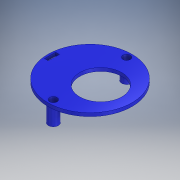
# Autodesk Inventor part: plate_r1
Saved by Autodesk Inventor 2018 (Build 220112000, 112)
## iProperties
Created: 2019-05-28
Part Number: plate_r1
Material: Generic
Document SubType Name: Modeling
Designer: Koki
Density: 1 g/cm^3
Appearance: Blue - Wall Paint - Glossy
Author: Koki
Autodesk Inventor part; units mm, degrees
ref_plane "YZ Plane" through (0, 0, 0) normal (1, 0, 0) x (0, 1, 0)
ref_plane "XZ Plane" through (0, 0, 0) normal (0, 1, 0) x (-1, 0, 0)
ref_plane "XY Plane" through (0, 0, 0) normal (0, 0, 1) x (1, 0, 0)
sketch "Sketch1" plane through (0, 0, 0) normal (0, 1, 0) x (-1, 0, 0)
  circle A0 centre (0, 0) radius 37.85
  dimension "d0" = 75.7
  constraints: 1 centre point, 1 coincident
  measures "d0" diameter of A0
extrude "Extrusion1" add sketch "Sketch1" along normal blind 3
sketch "Sketch2" plane through (0, 3, 0) normal (0, 1, 0) x (1, 0, 0)
  circle A0 centre (-33.02, 0) radius 3.4
  point P0 (0, 0)
  point P1 (0, 0)
  dimension "d3" = 33.02
  dimension "d4" = 6.8
  constraints: 1 centre point
  measures "d3" distance of point (0, 0) A0.centre
  measures "d4" diameter of A0
extrude "Extrusion2" cut sketch "Sketch2" against normal through all
mirror "Mirror1" about plane through (0, 0, 0) normal (1, 0, 0) of "Extrusion2"
sketch "Sketch3" plane through (0, 0, 0) normal (0, -1, 0) x (1, 0, 0)
  circle A0 centre (-33.02, 0) radius 3.4 projected
  circle A1 centre (33.02, 0) radius 3.4 projected
  circle A2 centre (-33.02, 0) radius 4.5
  circle A3 centre (33.02, 0) radius 4.5
  point P0 (0, 0)
  dimension "d7" = 9
  dimension "d8" = 9
  constraints: 2 centre point, 2 coincident
  measures "d7" diameter of A2
  measures "d8" diameter of A3
extrude "Extrusion3" add sketch "Sketch3" along normal blind 15
sketch "Sketch4" plane through (0, 3, 0) normal (0, 1, 0) x (1, 0, 0)
  circle A0 centre (0, -9.736) radius 19
  point P0 (0, 0)
  dimension "d11" = 9.736
  dimension "d12" = 38
  constraints: 1 centre point
  measures "d11" distance of A0.centre point (0, 0)
  measures "d12" diameter of A0
extrude "Extrusion4" cut sketch "Sketch4" against normal blind 18.5
sketch "Sketch5" plane through (0, 3, 0) normal (0, 1, 0) x (1, 0, 0)
  circle A0 centre (0, 8.554) radius 21
  point P0 (0, 0)
  dimension "d15" = 8.554
  dimension "d16" = 42
  constraints: 1 centre point
  measures "d15" distance of point (0, 0) A0.centre
  measures "d16" diameter of A0
extrude "Extrusion5" [suppressed]
sketch "Sketch6" plane through (0, 3, 0) normal (0, 1, 0) x (1, 0, 0)
  line L0 (5, 36) -> (-5, 36)
  line L1 (-5, 36) -> (-5, 32.5)
  line L2 (-5, 32.5) -> (5, 32.5)
  line L3 (5, 32.5) -> (5, 36)
  circle A0 centre (0, 0) radius 37.85 projected
  dimension "d19" = 10
  dimension "d20" = 5
  dimension "d21" = 3.5
  dimension "d22" = 36
  constraints: 8 end point, 2 parallel, 1 horizontal, 1 perpendicular
  measures "d19" distance of L0.start L0.end
  measures "d20" distance from line of point (0, 0) L3
  measures "d21" distance of L2.end L0.start
  measures "d22" distance from line of A0.centre L0
extrude "Extrusion6" cut sketch "Sketch6" against normal through all contours L3 L2 L1 L0
equation "\"d8\" = d7"
equation "\"d20\" = 0.5 * d19"
body "Solid1"
